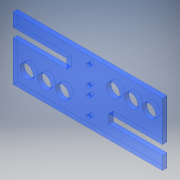
# Autodesk Inventor part: vexPlate
Saved by Autodesk Inventor 2016 SP1 (Build 200210100, 210)
## iProperties
Created: 2015-11-22
Part Number: vexPlate
Material: PET Plastic
Document SubType Name: Modeling
Designer: steele
Density: 1.541 g/cm^3
Appearance: Clear - Blue
Mass: 232.784 g
Surface Area: 544.371 cm^2
Volume: 151.06 cm^3
Author: steele
Autodesk Inventor part; units mm, degrees
ref_plane "YZ Plane" through (0, 0, 0) normal (1, 0, 0) x (0, 1, 0)
ref_plane "XZ Plane" through (0, 0, 0) normal (0, 1, 0) x (-1, 0, 0)
ref_plane "XY Plane" through (0, 0, 0) normal (0, 0, 1) x (1, 0, 0)
sketch "Sketch1" plane through (0, 0, 0) normal (0, 0, 1) x (1, 0, 0)
  line L0 (-105.918, -44.45) -> (105.918, -44.45)
  line L1 (105.918, -44.45) -> (105.918, 44.45)
  line L2 (105.918, 44.45) -> (-105.918, 44.45)
  line L3 (-105.918, 44.45) -> (-105.918, -44.45)
  line L4 (-29.718, 44.45) -> (-29.718, -44.45) construction
  line L5 (29.718, 44.45) -> (29.718, -44.45) construction
  line L6 (-105.918, 19.05) -> (105.918, 19.05) construction
  line L7 (-105.918, -19.05) -> (105.918, -19.05) construction
  line L8 (-67.818, 44.45) -> (-67.818, -44.45) construction
  line L9 (67.818, 44.45) -> (67.818, -44.45) construction
  line L10 (-105.918, 12.446) -> (-29.718, 12.446)
  line L11 (-29.718, 12.446) -> (-29.718, 25.654)
  line L12 (-29.718, 25.654) -> (-105.918, 25.654)
  line L13 (-105.918, 25.654) -> (-105.918, 12.446)
  line L14 (-105.918, 12.446) -> (-29.718, 25.654) construction
  line L15 (-29.718, 12.446) -> (-105.918, 25.654) construction
  line L16 (29.718, -25.654) -> (105.918, -25.654)
  line L17 (105.918, -25.654) -> (105.918, -12.446)
  line L18 (105.918, -12.446) -> (29.718, -12.446)
  line L19 (29.718, -12.446) -> (29.718, -25.654)
  line L20 (29.718, -25.654) -> (105.918, -12.446) construction
  line L21 (105.918, -25.654) -> (29.718, -12.446) construction
  point P0 (0, 0)
  point P1 (-67.818, 19.05)
  point P2 (67.818, -19.05)
  dimension "d2" = 29.718
  dimension "d3" = 29.718
  dimension "d4" = 19.05
  dimension "d5" = 19.05
  dimension "d6" = 67.818
  dimension "d7" = 67.818
  dimension "d9" = 13.208
  dimension "d10" = 76.2
  dimension "d11" = 105.918
  dimension "d12" = 44.45
  dimension "d15" = 105.918
  dimension "d16" = 44.45
  constraints: 44 end point, 16 point on line, 10 parallel, 9 perpendicular, 4 midpoint, 1 horizontal
  measures "d2" distance from line of L4 point (0, 0)
  measures "d3" distance from line of point (0, 0) L5
  measures "d4" distance from line of point (0, 0) L6
  measures "d5" distance from line of point (0, 0) L7
  measures "d6" distance from line of L8 point (0, 0)
  measures "d7" distance from line of point (0, 0) L9
  measures "d9" distance of L12.end L10.start
  measures "d10" distance of L11.end L12.end
  measures "d11" distance from line of point (0, 0) L3
  measures "d12" distance from line of point (0, 0) L2
  measures "d15" distance from line of point (0, 0) L1
  measures "d16" distance from line of point (0, 0) L0
extrude "Extrusion1" add sketch "Sketch1" against normal blind 6.35 contours L3 L10 L11 L12 L2 L1 L18 L19 L16 L0
sketch "Sketch2" plane through (0, 0, 0) normal (0, 0, 1) x (1, 0, 0)
  point P0 (0, 0)
  point P1 (0, 31.75)
  point P2 (0, 6.35)
  point P3 (0, -6.35)
  point P4 (0, -31.75)
  dimension "d17" = 25.4
  dimension "d18" = 6.35
  dimension "d19" = 6.35
  dimension "d20" = 25.4
  measures "d17" distance of point (0, -31.75) point (0, -6.35)
  measures "d18" distance of point (0, -6.35) point (0, 0)
  measures "d19" distance of point (0, 6.35) point (0, 0)
  measures "d20" distance of point (0, 31.75) point (0, 6.35)
hole "Hole1" at (0, 31.75, 0) at (0, 6.35, 0) at (0, -6.35, 0) at (0, -31.75, 0) direction (0, 0, -1) diameter 5.1054 end through all clearance for "Flat Head Machine Screw (82)" size "#10" standard "Ansi Unified Screw Threads"
sketch "Sketch4" plane through (0, 0, 0) normal (0, 0, 1) x (1, 0, 0)
  line L0 (-105.918, -44.45) -> (-105.918, 12.446) construction
  line L1 (-105.918, -19.05) -> (0, -19.05) construction
  circle A0 centre (-86.868, -19.05) radius 9.525
  circle A1 centre (-61.468, -19.05) radius 9.525
  circle A2 centre (-36.068, -19.05) radius 9.525
  line L2 (0, 19.05) -> (105.8361, 19.05) construction
  circle A3 centre (86.868, 19.05) radius 9.525
  line L3 (105.918, -12.446) -> (105.918, 44.45) projected
  circle A4 centre (61.468, 19.05) radius 9.525
  circle A5 centre (36.068, 19.05) radius 9.525
  point P0 (0, 0)
  dimension "d28" = 19.05
  dimension "d29" = 19.05
  dimension "d32" = 25.4
  dimension "d37" = 19.05
  dimension "d38" = 19.05
  dimension "d39" = 19.05
  dimension "d40" = 19.05
  dimension "d43" = 25.4
  constraints: 6 centre point, 4 end point, 4 horizontal, 3 point on line, 8 other
  measures "d28" diameter of A0
  measures "d29" distance of L1.start A0.centre
  measures "d32" distance of A0.centre A1.centre
  measures "d37" distance from line of L1 point (0, 0)
  measures "d38" distance from line of L2 point (0, 0)
  measures "d39" distance from line of A3.centre L3
  measures "d40" diameter of A3
  measures "d43" distance of A3.centre A4.centre
extrude "Extrusion2" cut sketch "Sketch4" against normal through all
equation "\"d2\" = offsetForBracketHoles"
equation "\"d3\" = offsetForBracketHoles"
equation "\"d4\" = verticalCenterLineOfSlot"
equation "\"d5\" = verticalCenterLineOfSlot"
equation "\"d6\" = horizontalCenterLineOfSlot"
equation "\"d7\" = horizontalCenterLineOfSlot"
equation "\"d9\" = slotWidth"
equation "\"d10\" = slotLength"
equation "\"d11\" = 0.5 * plateWidth"
equation "\"d12\" = 0.5 * plateHeight"
equation "\"d15\" = 0.5 * plateWidth"
equation "\"d16\" = 0.5 * plateHeight"
equation "\"d13\" = plateThickness"
equation "\"d17\" = boltCentersForBracket"
equation "\"d20\" = boltCentersForBracket"
equation "\"d37\" = verticalCenterLineOfSlot"
equation "\"d38\" = verticalCenterLineOfSlot"
equation "\"plateWidth\" = 2 * offsetForBracketHoles + 2 * slotLength + 2 * edgeForSlot"
equation "\"plateHeight\" = 88.9"
equation "\"offsetForBracketHoles\" = 29.718"
equation "\"slotLength\" = 76.2"
equation "\"verticalCenterLineOfSlot\" = 19.05"
equation "\"cylinderDiameter\" = 12.7"
equation "\"centerLineOfBracket\" = 17.526"
equation "\"horizontalCenterLineOfSlot\" = 0.5 * slotLength + offsetForBracketHoles"
equation "\"plateThickness\" = 6.35"
equation "\"edgeForSlot\" = 0"
equation "\"centerLineMiddleBracket\" = 14.224"
equation "\"boltCentersForBracket\" = 25.4"
equation "\"printerOffset\" = 0.508"
equation "\"slotWidth\" = 13.208"
body "Solid1"
